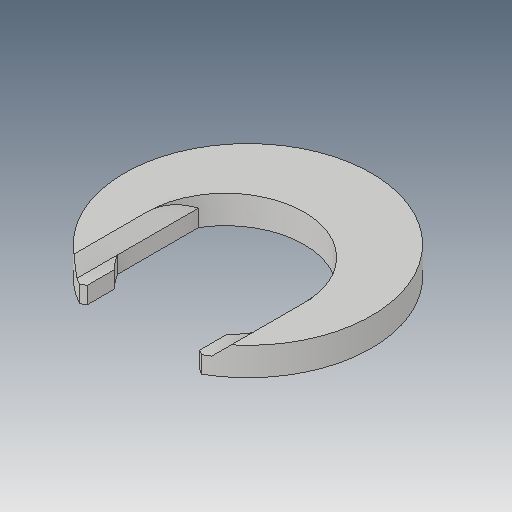
# Autodesk Inventor part: bottom_clip
Saved by Autodesk Inventor 2020.3 (Build 243373000, 373)
## iProperties
Created: 2021-02-25
Part Number: bottom_clip
Material: Generic
Document SubType Name: Modeling
Designer: paulg
Density: 1 g/cm^3
Appearance: Default
Author: paulg
Autodesk Inventor part; units mm, degrees
ref_plane "YZ Plane" through (0, 0, 0) normal (1, 0, 0) x (0, 1, 0)
ref_plane "XZ Plane" through (0, 0, 0) normal (0, 1, 0) x (-1, 0, 0)
ref_plane "XY Plane" through (0, 0, 0) normal (0, 0, 1) x (1, 0, 0)
sketch "Sketch1" plane through (0, 0, 0) normal (0, 0, 1) x (1, 0, 0)
  line L0 (0, 0) -> (-7, 0) construction
  line L1 (-7, 0) -> (-7, 2.5)
  line L2 (-7, 2.5) -> (-6, 1.5)
  line L3 (-6, 1.5) -> (-6, 0)
  line L4 (-7, 2.5) -> (-11, 2.5)
  line L5 (-11, 2.5) -> (-11, 0)
  line L6 (-11, 0) -> (-7, 0)
  line L7 (-7, 0) -> (-7, 2.5)
  line L8 (-7, 0) -> (-6, 0)
  dimension "d0" = 7
  dimension "d1" = 45
  dimension "d2" = 1
  dimension "d3" = 2.5
  dimension "d5" = 11
  constraints: 18 end point, 3 perpendicular, 2 collinear, 2 horizontal, 2 parallel, 1 point on line
  measures "d0" distance of L0.start L0.end
  measures "d1" angle of L1 L2
  measures "d2" distance between parallel lines of L1 L3
  measures "d3" distance of L0.end L1.end
  measures "d5" distance of L5.end L0.start
extrude "Extrusion1" add sketch "Sketch1" along normal mid plane 24
mirror "Mirror1" about plane through (0, 0, 0) normal (1, 0, 0) of "Extrusion1"
sketch "Sketch2" plane through (-11, 0, 12) normal (0, -1, 0) x (1, 0, 0)
  line L0 (5, -24) -> (5, 0) projected
  line L1 (0, 0) -> (5, 0) projected
  line L2 (0, -24) -> (0, 0) projected
  line L3 (5, -24) -> (0, -24) projected
  line L4 (17, -24) -> (17, 0) projected
  line L5 (17, -24) -> (22, -24) projected
  line L6 (22, -24) -> (22, 0) projected
  line L7 (22, 0) -> (17, 0) projected
  line L8 (11, -12) -> (11, -11)
  line L9 (5, -24) -> (5, 0) projected
  arc A0 (4, -11) -> (18, -11) centre (11, -11) ccw
  line L10 (11, -12) -> (11, -13)
  arc A1 (4, -21.4853) -> (18, -21.4853) centre (11, -13) ccw
  line L11 (17, -24) -> (17, 0) projected
  line L12 (4, 0) -> (4, -24) projected
  line L13 (18, 0) -> (18, -24) projected
  line L14 (4, -11) -> (4, -21.4853)
  line L15 (18, -11) -> (18, -21.4853)
  dimension "d8" = 1
  dimension "d11" = 7
  dimension "d12" = 11
  constraints: 8 end point, 4 point on circle, 4 point on line, 3 vertical, 2 centre point, 2 coincident, 2 collinear
  measures "d8" distance of L8.start L8.end
  measures "d11" radius of A0
  measures "d12" radius of A1
extrude "Extrusion2" add sketch "Sketch2" against normal up to surface (2.5 mm away) contours A1 L12 A0 L0 | L0 A0 L4 A1 | L4 A0 L13 A1
sketch "Sketch3" plane through (-11, 0, 12) normal (0, -1, 0) x (1, 0, 0)
  line L0 (5, -14.6056) -> (5, 0) projected
  line L1 (0, 0) -> (5, 0) projected
  line L2 (0, -24) -> (0, 0) projected
  line L3 (5, -24) -> (0, -24) projected
  line L4 (5, -24) -> (5, -22.2195) projected
  arc A0 (5, -22.2195) -> (17, -22.2195) centre (11, -13) ccw projected
  line L5 (17, -24) -> (17, -22.2195) projected
  line L6 (17, -24) -> (22, -24) projected
  line L7 (22, -24) -> (22, 0) projected
  line L8 (22, 0) -> (17, 0) projected
  line L9 (17, -14.6056) -> (17, 0) projected
  arc A1 (5, -14.6056) -> (17, -14.6056) centre (11, -11) ccw projected
  line L10 (5, -14.6056) -> (5, 0) projected
  arc A2 (5, -14.6056) -> (17, -14.6056) centre (11, -11) ccw projected
  line L11 (6, -6.101) -> (6, -2.3397)
  line L12 (16, -6.101) -> (16, -2.3397)
  arc A3 (17, -3) -> (16, -2.3397) centre (11, -11) ccw
  arc A4 (6, -2.3397) -> (5, -3) centre (11, -11) ccw
  arc A5 (17, -7.3944) -> (16, -6.101) centre (11, -11) ccw
  arc A6 (6, -6.101) -> (5, -7.3944) centre (11, -11) ccw
  line L13 (17, -3) -> (17, -7.3944)
  line L14 (17, -14.6056) -> (17, 0) projected
  line L15 (5, -3) -> (5, -7.3944)
  point P0 (11, -12)
  dimension "d15" = 1
  dimension "d16" = 1
  dimension "d17" = 10
  constraints: 8 end point, 8 point on circle, 4 centre point, 4 point on line, 3 concentric, 2 coincident, 2 collinear, 1 vertical
  measures "d15" distance between parallel lines of L11 L0
  measures "d16" distance between parallel lines of L9 L12
  measures "d17" radius of A4
extrude "Extrusion3" add sketch "Sketch3" against normal blind 1.5 contours L0 A4 L11 A6 | A5 L12 A3 L9
sketch "Sketch4" plane through (-11, 0, 12) normal (0, -1, 0) x (1, 0, 0)
  line L0 (5, -14.6056) -> (5, -7.3944) construction
  arc A0 (6, -6.101) -> (5, -7.3944) centre (11, -11) ccw construction
  line L1 (6, -6.101) -> (6, -2.3397) construction
  arc A1 (6, -2.3397) -> (5, -3) centre (11, -11) ccw construction
  line L2 (5, -3) -> (5, 0) construction
  line L3 (0, 0) -> (5, 0) construction
  line L4 (0, -24) -> (0, 0) construction
  line L5 (5, -24) -> (0, -24) construction
  line L6 (5, -24) -> (5, -22.2195) construction
  arc A2 (5, -22.2195) -> (17, -22.2195) centre (11, -13) ccw construction
  line L7 (17, -24) -> (17, -22.2195) construction
  line L8 (17, -24) -> (22, -24) construction
  line L9 (22, -24) -> (22, 0) construction
  line L10 (22, 0) -> (17, 0) construction
  line L11 (17, -3) -> (17, 0) construction
  arc A3 (17, -3) -> (16, -2.3397) centre (11, -11) ccw construction
  line L12 (16, -2.3397) -> (16, -6.101) construction
  arc A4 (17, -7.3944) -> (16, -6.101) centre (11, -11) ccw construction
  line L13 (17, -14.6056) -> (17, -7.3944) construction
  arc A5 (5, -14.6056) -> (17, -14.6056) centre (11, -11) ccw construction
  circle A6 centre (11, -13) radius 11
  circle A7 centre (11, -13) radius 19.3975
  point P0 (11, -12)
  constraints: 2 centre point, 2 coincident, 1 concentric
extrude "Extrusion4" cut sketch "Sketch4" against normal through all
chamfer "Chamfer1" distance 0.5 angle 45 2 edges at (-5, 0.75, 8.798) (5, 0.75, 8.798)
equation "\"d16\" = d15"
body "Solid1"
